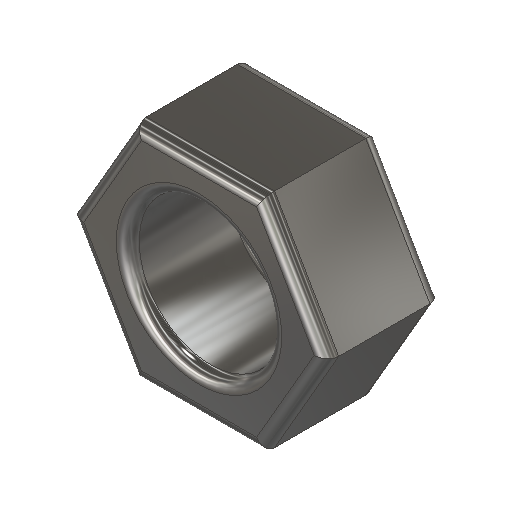
# Autodesk Inventor part: COTS_GENERIC_M5_Nut
Saved by Autodesk Inventor 2025 (Build 290162010, 162A)
## iProperties
Created: 2018-07-31
Part Number: COTS_GENERIC_M5_Nut
Material: Generic
Document SubType Name: Modeling
Designer: Andrzej
Density: 1 g/cm^3
Appearance: Steel - Polished
Author: Andrzej
Autodesk Inventor part; units mm, degrees
ref_plane "YZ Plane" through (0, 0, 0) normal (1, 0, 0) x (0, 1, 0)
ref_plane "XZ Plane" through (0, 0, 0) normal (0, 1, 0) x (-1, 0, 0)
ref_plane "XY Plane" through (0, 0, 0) normal (0, 0, 1) x (1, 0, 0)
sketch "Sketch1" plane through (0, 0, 0) normal (0, 0, 1) x (1, 0, 0)
  circle A0 centre (0, 0) radius 2.5
  circle A1 centre (0, 0) radius 3.9
  line L0 (2.2517, 3.9) -> (4.5033, 0)
  line L1 (4.5033, 0) -> (2.2517, -3.9)
  line L2 (2.2517, -3.9) -> (-2.2517, -3.9)
  line L3 (-2.2517, -3.9) -> (-4.5033, 0)
  line L4 (-4.5033, 0) -> (-2.2517, 3.9)
  line L5 (-2.2517, 3.9) -> (2.2517, 3.9)
  point P0 (0, 3.9)
  dimension "d1" = 7.8
  dimension "d0" = 5
  constraints: 12 end point, 3 coincident, 1 centre point, 1 midpoint, 1 vertical alignment, 15 other
  measures "d0" diameter of A0
extrude "Extrusion1" add sketch "Sketch1" along normal blind 4
fillet "Fillet1" radius 0.4 16 edges at (1.1258, 3.9, 4) (-1.1258, 3.9, 4) (-2.5, 0, 4) (-3.3775, 1.95, 4) (0, -3.9, 4) (-3.3775, -1.95, 4) (3.3775, -1.95, 4) (3.3775, 1.95, 4) (3.3775, 1.95, 0) (1.1258, 3.9, 0) (-1.1258, 3.9, 0) (3.3775, -1.95, 0) (0, -3.9, 0) (-2.5, 0, 0) (-3.3775, -1.95, 0) (-3.3775, 1.95, 0)
body "Solid1"
